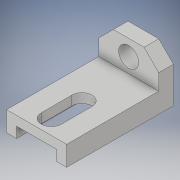
# Autodesk Inventor part: 410571040練習二
Saved by Autodesk Inventor 2017 (Build 210142000, 142)
## iProperties
Part Number: 410571040練習二
Material: 一般
Document SubType Name: Modeling
Designer: user
Density: 1 g/cm^3
Appearance: 預設
Author: user
Autodesk Inventor part; units mm, degrees
ref_plane "YZ Plane" through (0, 0, 0) normal (1, 0, 0) x (0, 1, 0)
ref_plane "XZ Plane" through (0, 0, 0) normal (0, 1, 0) x (-1, 0, 0)
ref_plane "XY Plane" through (0, 0, 0) normal (0, 0, 1) x (1, 0, 0)
sketch "草圖1" plane through (0, 0, 0) normal (0, 0, 1) x (1, 0, 0)
  line L0 (0, 0) -> (0, 15)
  line L1 (0, 15) -> (45, 15)
  line L2 (45, 15) -> (45, 0)
  line L3 (45, 0) -> (37.5, 0)
  line L4 (37.5, 0) -> (37.5, 8)
  line L5 (37.5, 8) -> (7.5, 8)
  line L6 (7.5, 8) -> (7.5, 0)
  line L7 (7.5, 0) -> (0, 0)
  dimension "d0" = 15
  dimension "d1" = 8
  dimension "d2" = 30
  dimension "d3" = 45
  dimension "d4" = 7.5
  constraints: 16 end point, 7 perpendicular, 1 point on line, 1 vertical
  measures "d0" distance of L0.start L0.end
  measures "d1" distance of L5.end L6.end
  measures "d2" distance of L4.end L5.end
  measures "d3" distance between parallel lines of L2 L0
  measures "d4" distance between parallel lines of L2 L4
extrude "擠出1" add sketch "草圖1" against normal blind 80
sketch "草圖2" plane through (0, 15, 0) normal (0, 1, 0) x (1, 0, 0)
  line L0 (15, 34) -> (15, 11)
  line L1 (30, 34) -> (30, 11)
  arc A0 (30, 34) -> (15, 34) centre (22.5, 34) ccw
  arc A1 (15, 11) -> (30, 11) centre (22.5, 11) ccw
  line L2 (0, 0) -> (45, 0) projected
  line L3 (0, 0) -> (0, 80) projected
  dimension "d7" = 11
  dimension "d8" = 15
  dimension "d9" = 7.5
  dimension "d10" = 23
  dimension "d11" = 7.5
  dimension "d12" = 22.5
  constraints: 4 end point, 4 point on circle, 2 centre point, 2 vertical
  measures "d7" distance from line of A1.centre L2
  measures "d8" distance between parallel lines of L1 L0
  measures "d9" radius of A1
  measures "d10" distance of A1.centre A0.centre
  measures "d11" radius of A0
  measures "d12" distance from line of A0.centre L3
extrude "擠出2" cut sketch "草圖2" against normal blind 7
sketch "草圖3" plane through (0, 0, -80) normal (0, 0, -1) x (-1, 0, 0)
  line L0 (-45, 15) -> (-45, 0) projected
  line L1 (-45, 15) -> (-45, 27)
  line L2 (-45, 27) -> (-34, 38)
  line L3 (-34, 38) -> (-11, 38)
  line L4 (-11, 38) -> (0, 27)
  line L5 (0, 27) -> (0, 15)
  line L6 (0, 15) -> (-45, 15) projected
  line L7 (0, 15) -> (-45, 15)
  circle A0 centre (-22.5, 26) radius 7.5
  line L8 (-7.5, 0) -> (0, 0) projected
  dimension "d15" = 11
  dimension "d16" = 11
  dimension "d17" = 11
  dimension "d18" = 11
  dimension "d19" = 38
  dimension "d20" = 11
  dimension "d21" = 15
  dimension "d22" = 22.5
  constraints: 12 end point, 2 perpendicular, 1 centre point, 1 parallel, 1 vertical
  measures "d15" horizontal distance of L4.end L3.end
  measures "d16" horizontal distance of L4.end L3.end
  measures "d17" horizontal distance of L2.end L1.end
  measures "d18" horizontal distance of L1.end L2.end
  measures "d19" distance between parallel lines of L8 L3
  measures "d20" distance from line of L6 A0.centre
  measures "d21" diameter of A0
  measures "d22" distance from line of L5 A0.centre
extrude "擠出3" add sketch "草圖3" against normal blind 11
